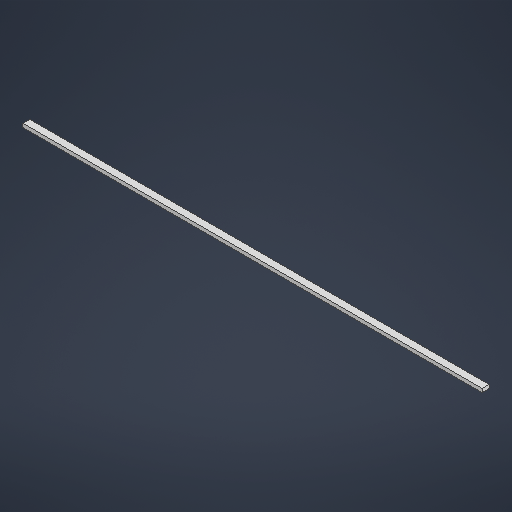
# Autodesk Inventor part: Rack
Saved by Autodesk Inventor 2026.1 (Build 301233020, 233B)
## iProperties
Created: 2026-03-11
Part Number: Rack
Material: Generic
Document SubType Name: Modeling
Designer: elaij
Density: 1 g/cm^3
Appearance: Default
Author: elaij
Autodesk Inventor part; units mm, degrees
ref_plane "YZ Plane" through (0, 0, 0) normal (1, 0, 0) x (0, 1, 0)
ref_plane "XZ Plane" through (0, 0, 0) normal (0, 1, 0) x (-1, 0, 0)
ref_plane "XY Plane" through (0, 0, 0) normal (0, 0, 1) x (1, 0, 0)
sketch "Sketch3" plane through (0, 0, 0) normal (1, 0, 0) x (0, 1, 0)
  line L0 (0, 0) -> (8, 0)
  line L1 (8, 0) -> (8, 15)
  line L2 (8, 15) -> (0, 15)
  line L3 (0, 15) -> (0, 0)
  dimension "d30" = 8
  dimension "d31" = 15
  constraints: 8 end point, 2 parallel, 1 horizontal, 1 perpendicular
  measures "d30" distance of L0.start L0.end
  measures "d31" distance between parallel lines of L0 L2
extrude "Extrusion3" add sketch "Sketch3" along normal blind 1000
equation "\"ToothCut\" = 3"
equation "\"Width\" = 6"
body "Solid2"
